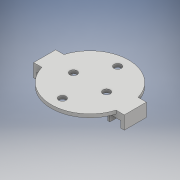
# Autodesk Inventor part: loadCelMount
Saved by Autodesk Inventor 2018 (Build 220112000, 112)
## iProperties
Created: 2018-05-09
Part Number: loadCelMount
Material: Generic
Document SubType Name: Modeling
Designer: s4321966
Density: 1 g/cm^3
Appearance: Default
Mass: 1.90902 g
Surface Area: 26.5149 cm^2
Volume: 1.90902 cm^3
Author: s4321966
Autodesk Inventor part; units mm, degrees
ref_plane "YZ Plane" through (0, 0, 0) normal (1, 0, 0) x (0, 1, 0)
ref_plane "XZ Plane" through (0, 0, 0) normal (0, 1, 0) x (-1, 0, 0)
ref_plane "XY Plane" through (0, 0, 0) normal (0, 0, 1) x (1, 0, 0)
sketch "Sketch1" plane through (0, 0, 0) normal (0, 0, 1) x (1, 0, 0)
  line L0 (0, 0) -> (4, 0)
  line L1 (4, 0) -> (4, 13)
  line L2 (4, 13) -> (0, 13)
  line L3 (0, 13) -> (0, 0)
  line L4 (4, 13) -> (-4, 13)
  line L5 (-4, 13) -> (-4, -8)
  line L6 (-4, -8) -> (4, -8)
  line L7 (4, -8) -> (4, 13)
  line L8 (-4, 13) -> (4, 13)
  line L9 (4, 13) -> (4, 21)
  line L10 (4, 21) -> (-4, 21)
  line L11 (-4, 21) -> (-4, 13)
  line L12 (4, 21) -> (7, 21)
  line L13 (7, 21) -> (7, 13)
  line L14 (7, 13) -> (4, 13)
  line L15 (4, 13) -> (4, 21)
  line L16 (7, 21) -> (11, 21)
  line L17 (11, 21) -> (11, 13)
  line L18 (11, 13) -> (7, 13)
  line L19 (7, 13) -> (7, 21)
  line L20 (11, 13) -> (4, 13)
  line L21 (4, 13) -> (4, -8)
  line L22 (4, -8) -> (11, -8)
  line L23 (4, -8) -> (11, -8)
  line L24 (11, -8) -> (11, 0)
  line L25 (11, 0) -> (4, 0)
  line L26 (4, 0) -> (4, -8)
  line L27 (11, -8) -> (14, -8)
  line L28 (14, -8) -> (14, 0)
  line L29 (14, 0) -> (11, 0)
  line L30 (11, 0) -> (11, -8)
  line L31 (14, -8) -> (19, -8)
  line L32 (19, -8) -> (19, 13)
  line L33 (19, 13) -> (14, 13)
  line L34 (14, 13) -> (14, -8)
  line L35 (14, 13) -> (22, 13)
  line L36 (14, 18) -> (14, 13)
  line L37 (19, 13) -> (14, 13)
  line L38 (14, 13) -> (14, 21)
  line L39 (14, 21) -> (19, 21)
  line L40 (19, 21) -> (19, 13)
  line L41 (19, -8) -> (-19, -8)
  line L42 (-19, -8) -> (-19, 0)
  line L43 (-19, 0) -> (19, 0)
  line L44 (19, 0) -> (19, -8)
  line L45 (-4, 0) -> (-7, 0)
  line L46 (-7, 0) -> (-7, -8)
  line L47 (-7, -8) -> (-4, -8)
  line L48 (-4, -8) -> (-4, 0)
  line L49 (-7, 0) -> (-11, 0)
  line L50 (-11, 0) -> (-11, -8)
  line L51 (-11, -8) -> (-7, -8)
  line L52 (-7, -8) -> (-7, 0)
  line L53 (-11, -8) -> (-14, -8)
  line L54 (-14, -8) -> (-14, 0)
  line L55 (-14, 0) -> (-11, 0)
  line L56 (-11, 0) -> (-11, -8)
  line L57 (7, 13) -> (11, 13)
  line L58 (11, 13) -> (11, 3)
  line L59 (11, 3) -> (7, 3)
  line L60 (7, 3) -> (7, 13)
  line L61 (-4, 13) -> (-7, 13)
  line L62 (-7, 13) -> (-7, 21)
  line L63 (-7, 21) -> (-4, 21)
  line L64 (-4, 21) -> (-4, 13)
  line L65 (-7, 21) -> (-11, 21)
  line L66 (-11, 21) -> (-11, 13)
  line L67 (-11, 13) -> (-7, 13)
  line L68 (-7, 13) -> (-7, 21)
  line L69 (-7, 13) -> (-11, 13)
  line L70 (-11, 13) -> (-11, 3)
  line L71 (-11, 3) -> (-7, 3)
  line L72 (-7, 3) -> (-7, 13)
  line L73 (-19, -8) -> (-14, -8)
  line L74 (-14, -8) -> (-14, 13)
  line L75 (-14, 13) -> (-19, 13)
  line L76 (-19, 13) -> (-19, -8)
  dimension "d0" = 4
  dimension "d1" = 13
  dimension "d2" = 8
  dimension "d3" = 21
  dimension "d4" = 8
  dimension "d5" = 8
  dimension "d6" = 3
  dimension "d7" = 8
  dimension "d8" = 4
  dimension "d9" = 8
  dimension "d10" = 3
  dimension "d11" = 8
  dimension "d12" = 5
  dimension "d13" = 21
  dimension "d16" = 5
  dimension "d17" = 8
  dimension "d18" = 38
  dimension "d19" = 8
  dimension "d20" = 3
  dimension "d21" = 8
  dimension "d22" = 4
  dimension "d23" = 8
  dimension "d24" = 3
  dimension "d25" = 8
  dimension "d26" = 10
  dimension "d27" = 3
  dimension "d28" = 8
  dimension "d29" = 4
  dimension "d30" = 8
  dimension "d31" = 4
  dimension "d32" = 10
  dimension "d33" = 5
  dimension "d34" = 21
  constraints: 154 end point, 37 parallel, 20 horizontal, 19 perpendicular, 2 point on line
  measures "d0" distance of L2.end L1.end
  measures "d1" distance of L1.end L0.end
  measures "d2" distance of L6.end L5.end
  measures "d3" distance of L5.end L4.end
  measures "d4" distance of L10.end L9.end
  measures "d5" distance of L9.end L8.end
  measures "d6" distance of L13.end L14.end
  measures "d7" distance of L12.end L13.end
  measures "d8" distance of L17.end L18.end
  measures "d9" distance of L16.end L17.end
  measures "d10" distance of L29.end L28.end
  measures "d11" distance of L28.end L27.end
  measures "d12" distance of L33.end L32.end
  measures "d13" distance of L32.end L31.end
  measures "d16" distance of L38.end L39.end
  measures "d17" distance of L37.end L38.end
  measures "d18" distance of L42.end L43.end
  measures "d19" distance of L41.end L42.end
  measures "d20" distance of L47.end L46.end
  measures "d21" distance of L46.end L45.end
  measures "d22" distance of L51.end L50.end
  measures "d23" distance of L50.end L49.end
  measures "d24" distance of L54.end L55.end
  measures "d25" distance of L53.end L54.end
  measures "d26" distance of L57.end L58.end
  measures "d27" distance of L62.end L63.end
  measures "d28" distance of L61.end L62.end
  measures "d29" distance of L67.end L66.end
  measures "d30" distance of L66.end L65.end
  measures "d31" distance of L71.end L70.end
  measures "d32" distance of L70.end L69.end
  measures "d33" distance of L75.end L74.end
  measures "d34" distance of L74.end L73.end
extrude "Extrusion1" add sketch "Sketch1" along normal blind 2.5 contours L3 L2 L1 L0 | L43 L5 L4 L3 | L0 L7 L6 L5 L43 | L25 L24 L22 L7 | L4 L11 L10 L9 L2 | L5 L41 L46 L43 | L9 L12 L13 L14 | L29 L28 L27 L24 | L61 L62 L63 L11 | L46 L41 L50 L43 | L13 L16 L17 L18 | L18 L58 L59 L60 | L43 L32 L31 L28 | L34 L33 L32 L43 | L67 L66 L65 L62 | L72 L71 L70 L67 | L50 L41 L54 L43 | L54 L41 L42 L43 | L43 L76 L75 L74
sketch "Sketch2" plane through (0, 0, 2.5) normal (0, 0, 1) x (1, 0, 0)
  line L0 (-14, 13) -> (-19, 13) projected
  line L1 (-19, 13) -> (-14, 13)
  line L2 (-14, 13) -> (-14, 8)
  line L3 (-14, 8) -> (-19, 8)
  line L4 (-19, 8) -> (-19, 13)
  line L5 (14, 13) -> (19, 13)
  line L6 (19, 13) -> (19, 8)
  line L7 (19, 8) -> (14, 8)
  line L8 (14, 8) -> (14, 13)
  line L9 (-20.5, 6.5) -> (-12.5, 6.5)
  line L10 (-12.5, 6.5) -> (-12.5, 14.5)
  line L11 (-12.5, 14.5) -> (-20.5, 14.5)
  line L12 (-20.5, 14.5) -> (-20.5, 6.5)
  line L13 (12.5, 6.5) -> (20.5, 6.5)
  line L14 (20.5, 6.5) -> (20.5, 14.5)
  line L15 (20.5, 14.5) -> (12.5, 14.5)
  line L16 (12.5, 14.5) -> (12.5, 6.5)
  line L17 (-20.5, 14.5) -> (-19, 14.5)
  line L18 (-19, 14.5) -> (-19, 4.5)
  line L19 (-19, 4.5) -> (-20.5, 4.5)
  line L20 (-20.5, 4.5) -> (-20.5, 14.5)
  line L21 (-14, 0) -> (-14, 13) projected
  line L22 (-12.5, 14.5) -> (-14, 14.5)
  line L23 (-14, 14.5) -> (-14, 4.5)
  line L24 (-14, 4.5) -> (-12.5, 4.5)
  line L25 (-12.5, 4.5) -> (-12.5, 14.5)
  line L26 (-19, 14.5) -> (-14, 14.5)
  line L27 (-14, 14.5) -> (-14, 13)
  line L28 (-14, 13) -> (-19, 13)
  line L29 (-19, 13) -> (-19, 14.5)
  line L30 (12.5, 14.5) -> (20.5, 14.5)
  line L31 (20.5, 14.5) -> (20.5, 13)
  line L32 (20.5, 13) -> (12.5, 13)
  line L33 (12.5, 13) -> (12.5, 14.5)
  line L34 (14, 13) -> (14, 0) projected
  line L35 (12.5, 14.5) -> (14, 14.5)
  line L36 (14, 14.5) -> (14, 4.5)
  line L37 (14, 4.5) -> (12.5, 4.5)
  line L38 (12.5, 4.5) -> (12.5, 14.5)
  line L39 (19, -8) -> (19, 13) projected
  line L40 (20.5, 14.5) -> (19, 14.5)
  line L41 (19, 14.5) -> (19, 4.5)
  line L42 (19, 4.5) -> (20.5, 4.5)
  line L43 (20.5, 4.5) -> (20.5, 14.5)
  point P0 (0, 0)
  dimension "d37" = 5
  dimension "d38" = 5
  dimension "d39" = 5
  dimension "d40" = 5
  dimension "d41" = 1.5
  dimension "d42" = 1.5
  dimension "d43" = 1.5
  dimension "d44" = 10
  dimension "d45" = 10
  dimension "d46" = 10
  constraints: 80 end point, 20 parallel, 10 perpendicular, 8 horizontal, 6 point on line, 6 other
  measures "d37" distance of L2.end L3.end
  measures "d38" distance of L1.end L2.end
  measures "d39" distance of L6.end L7.end
  measures "d40" distance of L5.end L6.end
  measures "d41" distance between parallel lines of L3 L9
  measures "d42" distance between parallel lines of L7 L13
  measures "d43" distance of L18.end L19.end
  measures "d44" distance of L17.end L18.end
  measures "d45" distance of L35.end L36.end
  measures "d46" distance of L41.end L40.end
extrude "Extrusion2" add sketch "Sketch2" along normal blind 3 contours L23 L11 L10 L9 L21 L2 | L0 L18 L11 L23 | L4 L18 L9 L12 L11 | L9 L25 L24 L21 | L18 L19 L20 L9 | L36 L15 L41 L5 | L8 L34 L13 L16 L32 | L32 L16 L15 L36 | L32 L14 L13 L39 L6 | L41 L15 L14 L32 | L34 L37 L38 L13 | L13 L43 L42 L39
sketch "Sketch4" plane through (0, 0, 5.5) normal (0, 0, 1) x (1, 0, 0)
  line L0 (-12.5, 14.5) -> (-20.5, 14.5) projected
  line L1 (-12.5, 4.5) -> (-12.5, 14.5) projected
  line L2 (-20.5, 14.5) -> (-12.5, 14.5)
  line L3 (-12.5, 14.5) -> (-12.5, 4.5)
  line L4 (-12.5, 4.5) -> (-20.5, 4.5)
  line L5 (-20.5, 4.5) -> (-20.5, 14.5)
  line L6 (12.5, 14.5) -> (12.5, 4.5) projected
  line L7 (20.5, 4.5) -> (20.5, 14.5) projected
  line L8 (12.5, 14.5) -> (20.5, 14.5)
  line L9 (20.5, 14.5) -> (20.5, 4.5)
  line L10 (20.5, 4.5) -> (12.5, 4.5)
  line L11 (12.5, 4.5) -> (12.5, 14.5)
  point P0 (0, 0)
  constraints: 16 end point, 4 parallel, 2 horizontal, 2 perpendicular
extrude "Extrusion3" add sketch "Sketch4" along normal blind 1.5
sketch "Sketch5" plane through (0, 0, 7) normal (0, 0, 1) x (1, 0, 0)
  line L0 (-12.5, 14.5) -> (-20.5, 14.5) projected
  line L1 (20.5, 4.5) -> (20.5, 14.5) projected
  line L2 (-20.5, 14.5) -> (20.5, 14.5)
  line L3 (20.5, 14.5) -> (20.5, 4.5)
  line L4 (20.5, 4.5) -> (-20.5, 4.5)
  line L5 (-20.5, 4.5) -> (-20.5, 14.5)
  line L6 (-20.5, 14.5) -> (-20.5, 4.5) projected
  line L7 (-20.5, 9.5) -> (20.5, 9.5)
  line L8 (0, 9.5) -> (0, 14.5)
  circle A0 centre (0, 9.5) radius 17.5
  point P0 (0, 0)
  constraints: 12 end point, 4 midpoint, 2 parallel, 1 centre point, 1 coincident, 1 horizontal, 1 perpendicular
extrude "Extrusion4" add sketch "Sketch5" along normal blind 1.5
sketch "Sketch6" plane through (0, 0, 8.5) normal (0, 0, 1) x (1, 0, 0)
  arc A0 (16.7705, 14.5) -> (-16.7705, 14.5) centre (0, 9.5) ccw projected
  circle A1 centre (0, 9.5) radius 17.5
  circle A2 centre (0, 9.5) radius 7.5
  circle A3 centre (0, 9.5) radius 12.5
  line L0 (12.5, 14.5) -> (12.5, 4.5) projected
  circle A4 centre (0, 9.5) radius 10
  circle A5 centre (0, -0.5) radius 1.651
  circle A6 centre (0, 2) radius 1.651
  circle A7 centre (7.5, 9.5) radius 1.651
  circle A8 centre (-7.5, 9.5) radius 1.651
  circle A9 centre (0, 17) radius 1.651
  circle A10 centre (0, 22) radius 1.651
  circle A11 centre (0, -3) radius 1.651
  point P0 (0, 0)
  dimension "d54" = 20
  dimension "d53" = 15
  dimension "d55" = 3.302
  dimension "d56" = 3.302
  dimension "d57" = 3.302
  dimension "d58" = 3.302
  dimension "d59" = 3.302
  dimension "d62" = 3.302
  dimension "d63" = 3.302
  constraints: 9 centre point, 6 point on circle, 4 coincident, 1 tangent, 1 vertical alignment, 5 other
  measures "d53" diameter of A2
  measures "d55" diameter of A5
  measures "d56" diameter of A6
  measures "d57" diameter of A7
  measures "d58" diameter of A8
  measures "d59" diameter of A9
  measures "d62" diameter of A10
  measures "d63" diameter of A11
extrude "Extrusion5" cut sketch "Sketch6" against normal blind 2.5 contours A2 A7 | A2 A7 | A8 A2 | A2 A8 | A11 A5 | A5 A11 A3 | A3 A11 | A10 A3 | A3 A10
sketch "Sketch7" plane through (0, 0, 2.5) normal (0, 0, -1) x (-1, 0, 0)
  line L0 (-36.0395, -19.2499) -> (42.4279, -19.2499)
  line L1 (42.4279, -19.2499) -> (42.4279, 35.743)
  line L2 (42.4279, 35.743) -> (-36.0395, 35.743)
  line L3 (-36.0395, 35.743) -> (-36.0395, -19.2499)
  point P0 (0, 0)
  constraints: 8 end point, 2 parallel, 1 horizontal, 1 perpendicular
extrude "Extrusion6" cut sketch "Sketch7" along normal blind 2.5
sketch "Sketch8" plane through (0, 0, 2.5) normal (0, 0, -1) x (-1, 0, 0)
  line L0 (-12.5, 14.5) -> (-12.5, 4.5) projected
  line L1 (-12.5, 14.5) -> (-13, 14.5)
  line L2 (-13, 14.5) -> (-13, 4.5)
  line L3 (-13, 4.5) -> (-12.5, 4.5)
  line L4 (-12.5, 4.5) -> (-12.5, 14.5)
  line L5 (12.5, 4.5) -> (12.5, 14.5) projected
  line L6 (12.5, 14.5) -> (13, 14.5)
  line L7 (13, 14.5) -> (13, 4.5)
  line L8 (13, 4.5) -> (12.5, 4.5)
  line L9 (12.5, 4.5) -> (12.5, 14.5)
  point P0 (0, 0)
  dimension "d66" = 0.5
  dimension "d67" = 10
  dimension "d68" = 0.5
  dimension "d69" = 10
  constraints: 16 end point, 4 parallel, 2 horizontal, 2 perpendicular
  measures "d66" distance of L3.end L2.end
  measures "d67" distance of L2.end L1.end
  measures "d68" distance of L7.end L8.end
  measures "d69" distance of L6.end L7.end
extrude "Extrusion7" cut sketch "Sketch8" against normal blind 4.5
body "Solid1"
